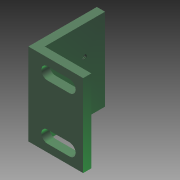
# Autodesk Inventor part: 13_0204_067
Saved by Autodesk Inventor 2012 SP1 (Build 160190100, 190)
## iProperties
Created: 2013-04-30
Part Number: 13_0204_067
Material: Default
Document SubType Name: Modeling
Designer: vogel
Density: 1 g/cm^3
Author: vogel
Autodesk Inventor part; units mm, degrees
ref_plane "YZ Plane" through (0, 0, 0) normal (1, 0, 0) x (0, 1, 0)
ref_plane "XZ Plane" through (0, 0, 0) normal (0, 1, 0) x (-1, 0, 0)
ref_plane "XY Plane" through (0, 0, 0) normal (0, 0, 1) x (1, 0, 0)
sketch "Skizze1" plane through (0, 0, 0) normal (0, 0, 1) x (1, 0, 0)
  line L0 (3, 3) -> (3, 25)
  line L1 (3, 25) -> (0, 25)
  line L2 (0, 25) -> (0, 0)
  line L3 (3, 3) -> (20, 3)
  line L4 (20, 3) -> (20, 0)
  line L5 (20, 0) -> (0, 0)
  dimension "d0" = 25
  dimension "d1" = 20
  dimension "d2" = 3
  constraints: 12 end point, 3 parallel, 2 perpendicular, 1 horizontal, 1 vertical
  measures "d0" distance between parallel lines of L1 L5
  measures "d1" distance of L4.end L2.end
  measures "d2" distance of L3.end L4.end
extrude "Extrusion1" add sketch "Skizze1" along normal blind 30
sketch "Skizze2" plane through (0, 0, 0) normal (0, -1, 0) x (1, 0, 0)
  line L0 (20, 30) -> (0, 30) projected
  line L1 (0, 0) -> (0, 30) projected
  line L2 (20, 0) -> (0, 0) projected
  line L3 (20, 0) -> (20, 30) projected
  line L4 (10, 30) -> (10, 0)
  line L5 (0, 15) -> (20, 15)
  point P0 (10, 25)
  point P1 (10, 5)
  dimension "d5" = 20
  dimension "d6" = 10
  constraints: 4 end point, 4 midpoint, 2 point on line, 1 parallel, 1 symmetric about line
  measures "d5" distance of point (10, 5) point (10, 25)
  measures "d6" distance between parallel lines of L4 L3
hole "Bohrung1" at (10, 0, 25) at (10, 0, 5) direction (0, 1, 0) diameter 4.5 end through all
sketch "Skizze3" plane through (3, 3, 0) normal (0, 1, 0) x (1, 0, 0)
  circle A0 centre (7, -25) radius 2.25 projected
  line L0 (17, 0) -> (17, -30) projected
  line L1 (4, -22.75) -> (12, -22.75)
  line L2 (12, -27.25) -> (4, -27.25)
  arc A1 (4, -22.75) -> (4, -27.25) centre (4, -25) ccw
  arc A2 (12, -27.25) -> (12, -22.75) centre (12, -25) ccw
  point P0 (-3, 0)
  dimension "d14" = 5
  dimension "d15" = 8
  constraints: 6 tangent, 4 end point, 4 point on circle, 2 centre point, 1 horizontal, 1 parallel
  measures "d14" distance from line of A2.centre L0
  measures "d15" distance of A1.centre A2.centre
extrude "Extrusion2" cut sketch "Skizze3" against normal through all contours A0 L1 A2 L2 | A0 L2 A1 L1
pattern_linear "Rechteckige Anordnung1" count 2 spacing 20 along (0, 0, -1) of "Extrusion2"
sketch "Skizze4" plane through (0, 0, 0) normal (-1, 0, 0) x (0, 0, 1)
  circle A0 centre (10, 17.5) radius 1.1 projected
  circle A1 centre (19.4, 17.5) radius 1.1 projected
  constraints: 2 coincident
hole "Bohrung2" at (0, 17.5, 10) at (0, 17.5, 19.4) direction (1, 0, 0) diameter 1.567 end through all thread size "M2x0.4" class "6H" standard "ISO Metric profile"
